Distanzen_v2 (Autodesk Fusion 360 design; units mm, degrees)
Autodesk Fusion 360 part; units mm, degrees
cylinder "Grundkörper Zylinder1" add diameter 8 height 10.2 placed x (1, 0, 0) y (0, 0, -1) z (0, 1, 0) at (0, 0, 0) makes body 1
cylinder "Grundkörper Zylinder2" cut diameter 3.2 height -19 placed x (1, 0, 0) y (0, 0, -1) z (0, 1, 0) at (0, 10.2, 0) bodies 1
copy_body "Körper->Berechn1" bodies 1 removing the originals makes body 2 in component "Component"
extrude "Extrusion1" add 1 faces at (3.1851, 10.2, 0.1987) along direction (0, 1, 0) blind 2.5 on bodies 2 bodies 2 in component "Component"
extrude "Extrusion2" add 1 faces at (3.1851, 12.7, 0.1987) along direction (0, 1, 0) blind 2.5 on bodies 2 bodies 2 in component "Component"
extrude "Extrusion3" cut 1 faces at (3.1792, 15.2, 0.2782) along direction (0, -1, 0) blind 7.5 on bodies 2 bodies 2 in component "Component"
extrude "Extrusion4" add 1 faces at (3.1851, 7.7, 0.1987) along direction (0, 1, 0) blind 2.5 on bodies 2 bodies 2 in component "Component"
component "Component" placed x (1, 0, 0) y (0, 1, 0) z (0, 0, 1) at (0, 0, 0)
